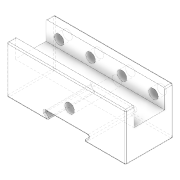
# Autodesk Inventor part: Turning and Facing Holder
Saved by Autodesk Inventor 2016 (Build 200138000, 138)
## iProperties
Created: 2020-10-21
Part Number: Turning and Facing Holder
Material: Generic
Document SubType Name: Modeling
Designer: extract
Density: 1 g/cm^3
Appearance: Default
Author: extract
Autodesk Inventor part; units mm, degrees
ref_plane "YZ Plane" through (0, 0, 0) normal (1, 0, 0) x (0, 1, 0)
ref_plane "XZ Plane" through (0, 0, 0) normal (0, 1, 0) x (-1, 0, 0)
ref_plane "XY Plane" through (0, 0, 0) normal (0, 0, 1) x (1, 0, 0)
sketch "Sketch1" plane through (0, 0, 0) normal (0, 1, 0) x (-1, 0, 0)
  line L0 (26.4286, 13.8687) -> (-23.5714, 13.8687)
  line L1 (-23.5714, 13.8687) -> (-23.5714, -6.1313)
  line L2 (-23.5714, -6.1313) -> (-5.5714, -6.1313)
  line L3 (-5.5714, -6.1313) -> (-8.5714, -3.1313)
  line L4 (-8.5714, -3.1313) -> (11.4286, -3.1313)
  line L5 (11.4286, -3.1313) -> (8.4286, -6.1313)
  line L6 (8.4286, -6.1313) -> (26.4286, -6.1313)
  line L7 (26.4286, -6.1313) -> (26.4286, 13.8687)
  point P0 (0, 0)
  dimension "d0" = 50
  dimension "d15" = 20
  dimension "d16" = 3
  dimension "d17" = 45
  dimension "d22" = 20
  constraints: 16 end point, 3 perpendicular, 2 equal length, 2 point on line, 1 horizontal, 1 parallel
  measures "d0" distance of L0.start L0.end
  measures "d15" distance between parallel lines of L6 L0
  measures "d16" distance between parallel lines of L6 L4
  measures "d17" angle of L6 L5
  measures "d22" distance of L3.end L4.end
extrude "Extrusion1" add sketch "Sketch1" along normal blind 20
sketch "Sketch2" plane through (23.5714, 0, 13.8687) normal (1, 0, 0) x (0, 0, -1)
  line L0 (0, 0) -> (0, 20) projected
  line L1 (0, 16.5) -> (8, 16.5)
  line L2 (8, 16.5) -> (8, 3.5)
  line L3 (8, 3.5) -> (0, 3.5)
  line L4 (0, 3.5) -> (0, 16.5)
  line L5 (0, 20) -> (20, 20) projected
  line L6 (5.2007, 20) -> (5.2007, 16.5) construction
  line L7 (5.2007, 3.5) -> (5.2007, 0) construction
  line L8 (0, 0) -> (20, 0) projected
  point P0 (13.8687, 0)
  dimension "d5" = 8
  dimension "d6" = 13
  constraints: 12 end point, 7 point on line, 2 parallel, 2 perpendicular, 1 collinear, 1 horizontal
  measures "d5" distance of L1.start L1.end
  measures "d6" distance of L1.end L2.end
extrude "Extrusion2" cut sketch "Sketch2" against normal through all
sketch "Sketch3" plane through (0, 20, 0) normal (0, 1, 0) x (1, 0, 0)
  circle A0 centre (-20.9015, -9.3037) radius 2
  circle A1 centre (-7.6759, -9.3037) radius 2
  circle A2 centre (5.5497, -9.3037) radius 2
  circle A3 centre (18.7753, -9.3037) radius 2
  line L0 (-20.9015, -9.3037) -> (-7.6759, -9.3037) construction
  line L1 (-7.6759, -9.3037) -> (5.5497, -9.3037) construction
  line L2 (5.5497, -9.3037) -> (18.7753, -9.3037) construction
  point P0 (0, 0)
  dimension "d9" = 4
  dimension "d10" = 4
  dimension "d11" = 4
  dimension "d12" = 4
  constraints: 6 end point, 4 centre point, 4 collinear, 1 horizontal
  measures "d9" diameter of A0
  measures "d10" diameter of A1
  measures "d11" diameter of A2
  measures "d12" diameter of A3
extrude "Extrusion3" cut sketch "Sketch3" against normal blind 5
fillet "Fillet1" radius 0.5 26 edges at (-26.4286, 18.25, 13.8687) (-26.4286, 20, 3.8687) (-26.4286, 10, -6.1313) (-26.4286, 0, 3.8687) (-26.4286, 1.75, 13.8687) (23.5714, 18.25, 13.8687) (-1.4286, 20, 13.8687) (23.5714, 1.75, 13.8687) (23.5714, 0, 3.8687) (23.5714, 10, -6.1313) (23.5714, 20, 3.8687) (-17.4286, 0, -6.1313) (-17.4286, 20, -6.1313) (-8.4286, 10, -6.1313) (-9.9286, 0, -4.6313) (-9.9286, 20, -4.6313) (-11.4286, 10, -3.1313) (-1.4286, 0, -3.1313) (-1.4286, 20, -3.1313) (8.5714, 10, -3.1313) (7.0714, 0, -4.6313) (7.0714, 20, -4.6313) (5.5714, 10, -6.1313) (14.5714, 0, -6.1313) (14.5714, 20, -6.1313) (-1.4286, 0, 13.8687)
sketch "Sketch4" plane through (0, 20, 0) normal (0, 1, 0) x (1, 0, 0)
  circle A0 centre (0, -2.9802) radius 2
  point P0 (0, 0)
  dimension "d19" = 4
  constraints: 1 centre point
  measures "d19" diameter of A0
extrude "Extrusion4" cut sketch "Sketch4" against normal through all
body "Solid1"
